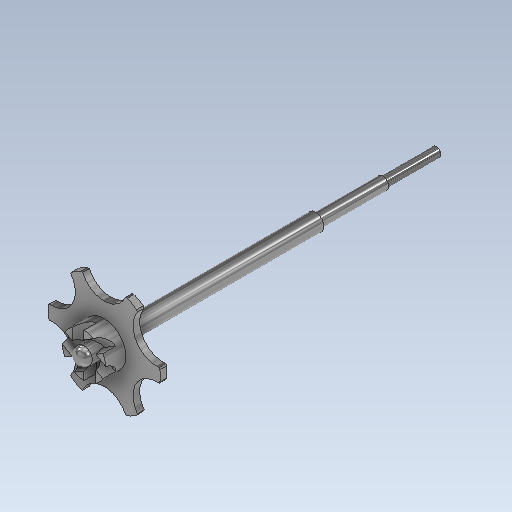
# Autodesk Inventor part: Baril do revólver
Saved by Autodesk Inventor 2021 (Build 250183000, 183)
## iProperties
Created: 2020-10-30
Part Number: Baril do revólver
Material: Liga de Nickel-Copper 400
Document SubType Name: Modeling
Designer: Bruno
Density: 8.83 g/cm^3
Appearance: Cromado - Preto polido
Author: Bruno
Autodesk Inventor part; units mm, degrees
sketch "Esboço1" plane through (0, 0, 0) normal (0, 0, 1) x (1, 0, 0)
  circle A0 centre (0, 0) radius 13
  dimension "d0" = 26
  constraints: 1 centre point, 1 coincident
  measures "d0" diameter of A0
extrude "Extrusão1" add sketch "Esboço1" against normal blind 33
sketch "Esboço2" plane through (0, 0, 0) normal (0, 0, 1) x (1, 0, 0)
  circle A0 centre (0, 0) radius 3.25
  dimension "d3" = 6.5
  constraints: 1 centre point, 1 coincident
  measures "d3" diameter of A0
sketch "Esboço3" plane through (0, 0, 0) normal (0, 0, 1) x (1, 0, 0)
  circle A0 centre (0, 8) radius 3.5
  point P0 (0, 0)
  dimension "d4" = 7
  dimension "d5" = 8
  constraints: 1 centre point
  measures "d4" diameter of A0
  measures "d5" distance of point (0, 0) A0.centre
extrude "Extrusão2" cut sketch "Esboço3" against normal through all
pattern_circular "Padrão circular1" count 6 over 360 about axis through (0, 0, 0) along (0, 0, -1) of "Extrusão2"
sketch "Esboço4" plane through (0, 0, -33) normal (0, 0, -1) x (-1, 0, 0)
  circle A0 centre (0, 0) radius 13 projected
  arc A1 (-9.1166, 9.2676) -> (-3.5411, 12.5084) centre (-6.533, 11.2392) ccw
  circle A2 centre (-6.9282, 4) radius 3.5 projected
  dimension "d11" = 6.5
  dimension "d12" = 0.5
  constraints: 5 point on circle, 1 centre point
  measures "d11" diameter of A1
extrude "Extrusão3" cut sketch "Esboço4" against normal blind 22 contours A1 A0 picked at (-5.9734, 10.2765)
sketch "Esboço6" plane through (0, 0, -11) normal (0, 0, -1) x (-1, 0, 0)
  arc A0 (-3.5411, 12.5084) -> (-9.1166, 9.2676) centre (0, 0) ccw projected
  arc A1 (-9.1166, 9.2676) -> (-3.5411, 12.5084) centre (-6.533, 11.2392) ccw projected
  arc A2 (-6.533, 7.9892) -> (-6.533, 14.4892) centre (-6.533, 11.2392) ccw
  line L0 (-6.533, 11.2392) -> (-6.533, 14.4892)
  line L1 (-6.533, 11.2392) -> (-6.533, 7.9892)
  arc A3 (-9.1166, 9.2676) -> (-3.5411, 12.5084) centre (-6.533, 11.2392) ccw projected
  point P0 (-3.5411, 12.5084)
  constraints: 4 end point, 4 point on circle, 1 centre point, 1 coincident, 1 point on line, 1 vertical
revolve "Revolução1" cut sketch "Esboço6" angle 360 about axis through (6.533, 11.2392, -11) along (0, 1, 0) picked at (-5.4827, 10.6075) contours A1 L1 A0 | A0 L0 A2
pattern_circular "Padrão circular2" count 6 over 360 about axis through (0, 0, -10) along (0, 0, 1) of "Extrusão3", "Revolução1"
ref_plane "Plano de trabalho2" through (0, 13, 0) normal (0, 1, 0) x (-1, 0, 0)
sketch "Esboço7" plane through (0, 13, 0) normal (0, 1, 0) x (-1, 0, 0)
  line L0 (1.75, -11.5) -> (-1.75, -11.5)
  line L1 (-1.75, -11.5) -> (-1.75, -4)
  line L2 (-1.75, -4) -> (1.75, -4)
  line L3 (1.75, -4) -> (1.75, -11.5)
  line L4 (1.75, -11.5) -> (-1.75, -4) construction
  line L5 (-1.75, -11.5) -> (1.75, -4) construction
  line L6 (13, 0) -> (-13, 0) projected
  point P0 (0, 0)
  point P1 (0, -7.75)
  dimension "d20" = 7.5
  dimension "d21" = 3.5
  dimension "d22" = 4
  constraints: 12 end point, 2 midpoint, 2 parallel, 1 horizontal, 1 perpendicular
  measures "d20" distance of L0.end L1.end
  measures "d21" distance of L1.end L2.end
  measures "d22" distance between parallel lines of L6 L2
extrude "Extrusão4" cut sketch "Esboço7" against normal blind 1
pattern_circular "Padrão circular3" count 6 over 360 about axis through (0, 0, -10) along (0, 0, 1) of "Extrusão4"
extrude "Extrusão5" add sketch "Esboço2" along normal blind 3
ref_plane "Plano de trabalho3" through (0, 3.25, 0) normal (0, 1, 0) x (-1, 0, 0)
sketch "Esboço8" plane through (0, 3.25, 0) normal (0, 1, 0) x (-1, 0, 0)
  line L0 (3.25, 3) -> (-3.25, 3) projected
  line L1 (0, 3) -> (0, 1.129)
  line L2 (13, 0) -> (-13, 0) projected
  arc A0 (0, 1.129) -> (1.7648, 3) centre (-0.4083, 3.2819) ccw
  point P0 (0, 0)
  dimension "d33" = 3.2819
  dimension "d34" = 2.1913
  dimension "d35" = 0.4083
  constraints: 2 end point, 2 point on circle, 1 centre point, 1 midpoint, 1 point on line, 1 vertical
  measures "d33" distance from line of L2 A0.centre
  measures "d34" radius of A0
  measures "d35" distance from line of L1 A0.centre
extrude "Extrusão6" cut sketch "Esboço8" against normal blind 3
pattern_circular "Padrão circular4" count 6 over 360 about axis through (0, 0, -10) along (0, 0, 1) of "Extrusão6"
sketch "Esboço9" plane through (0, 0, 3) normal (0, 0, 1) x (1, 0, 0)
  circle A0 centre (0, 0) radius 1.25
  dimension "d41" = 2.5
  constraints: 1 centre point, 1 coincident
  measures "d41" diameter of A0
extrude "Extrusão7" cut sketch "Esboço9" against normal through all
sketch "Esboço10" plane through (0, 0, 0) normal (0, 0, 1) x (1, 0, 0)
  circle A0 centre (0, 0) radius 8.35
  circle A1 centre (0, 0) radius 13
  dimension "d44" = 16.7
  constraints: 2 centre point, 2 coincident
  measures "d44" diameter of A0
extrude "Extrusão8" cut sketch "Esboço10" against normal through all
ref_plane "Plano de trabalho4" through (0, 0, -1) normal (0, 0, 1) x (1, 0, 0)
sketch "Esboço11" plane through (0, 0, -1) normal (0, 0, 1) x (1, 0, 0)
  circle A0 centre (0, 0) radius 1.25 projected
  circle A1 centre (0, 0) radius 8.35
  dimension "d48" = 16.7
  constraints: 1 centre point, 1 coincident
  measures "d48" diameter of A1
extrude "Extrusão9" cut sketch "Esboço11" against normal through all
ref_plane "Plano de trabalho5" through (0, 0, 3) normal (0, 0, 1) x (1, 0, 0)
sketch "Esboço12" plane through (0, 0, 3) normal (0, 0, 1) x (1, 0, 0)
  circle A0 centre (0, 0) radius 3.25 projected
  arc A1 (0, -1.25) -> (0, 1.25) centre (0, 0) ccw
  line L0 (0, 3.25) -> (0, 1.25) projected
  line L1 (0, 2.0975) -> (0, -2.2235)
  point P0 (1.0825, -0.625)
  constraints: 3 point on circle, 3 point on line, 2 end point, 1 centre point, 1 coincident, 1 collinear, 1 vertical alignment
revolve "Revolução2" add sketch "Esboço12" angle 360 about axis through (0, 2.0975, 3) along (0, -1, 0) contours L1 A1
sketch "Esboço13" plane through (0, 0, -1) normal (0, 0, -1) x (-1, 0, 0)
  circle A0 centre (0, 0) radius 1.25
  constraints: 1 centre point, 1 coincident
extrude "Extrusão10" add sketch "Esboço13" along normal blind 40.5 and the other way blind 4
sketch "Esboço14" plane through (0, 0, 0) normal (0, 0, 1) x (1, 0, 0)
  circle A0 centre (-4.3, 0) radius 0.25
  point P0 (0, 0)
  dimension "d57" = 0.5
  dimension "d58" = 4.3
  constraints: 1 centre point
  measures "d57" diameter of A0
  measures "d58" distance of point (0, 0) A0.centre
extrude "Extrusão11" cut sketch "Esboço14" against normal through all
sketch "Esboço15" plane through (0, 0, -41.5) normal (0, 0, -1) x (-1, 0, 0)
  circle A0 centre (0, 0) radius 0.9
  circle A1 centre (0, 0) radius 1.25
  dimension "d61" = 1.8
  dimension "d62" = 2.5
  constraints: 2 centre point, 2 coincident
  measures "d61" diameter of A0
  measures "d62" diameter of A1
extrude "Extrusão12" cut sketch "Esboço15" against normal blind 10
sketch "Esboço16" plane through (0, 0, -41.5) normal (0, 0, -1) x (-1, 0, 0)
  circle A0 centre (0, 0) radius 0.7
  dimension "d65" = 1.4
  constraints: 1 centre point, 1 coincident
  measures "d65" diameter of A0
extrude "Extrusão13" add sketch "Esboço16" along normal blind 8
thread "Rosca1" size "M1.4x0.3" class "6g" standard "ANSI Metric M Profile" length 15.255
sketch "Esboço17" plane through (0, 0, 0) normal (0, 0, 1) x (1, 0, 0)
  arc A0 (-3.4761, 7.592) -> (3.4761, 7.592) centre (0, 8) ccw projected
  arc A1 (-3.4761, 7.592) -> (3.4761, 7.592) centre (0, 8) ccw
  arc A2 (-3.4761, 7.592) -> (-4.8368, 6.8064) centre (0, 0) ccw projected
  line L0 (-3.4761, 7.592) -> (3.4761, 7.592)
  constraints: 2 end point, 2 point on circle, 1 centre point, 1 horizontal
extrude "Extrusão14" add sketch "Esboço17" against normal blind 1
sketch "Esboço18" plane through (0, 0, 0) normal (0, 0, 1) x (1, 0, 0)
  line L0 (-3.4761, 7.592) -> (3.4761, 7.592) projected
  circle A0 centre (0, 9) radius 3.5
  point P0 (0, 0)
  point P1 (3.2043, 7.592)
  point P2 (-3.2043, 7.592)
  dimension "d73" = 7
  dimension "d74" = 9
  constraints: 1 centre point
  measures "d73" diameter of A0
  measures "d74" distance of point (0, 0) A0.centre
extrude "Extrusão15" cut sketch "Esboço18" against normal blind 1 contours L0 A0 picked at (-0.0543, 6.4983)
pattern_circular "Padrão circular5" count 6 over 360 about axis through (0, 0, -10) along (0, 0, 1) of "Extrusão14", "Extrusão15"
